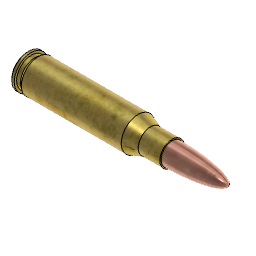
7-62x51mm_FMJ_mk1_v1 (Autodesk Fusion 360 design; units mm, degrees)
Autodesk Fusion 360 part; units mm, degrees
sketch "スケッチ1" plane through (0, 0, 0) normal (0, 0, 1) x (1, 0, 0)
  line L0 (0, 0) -> (71.12, 0)
  line L1 (0.458, 6.007) -> (0.458, -6.007) construction
  line L2 (0, 5.549) -> (0, -5.549)
  line L3 (0.458, 6.007) -> (0, 5.549)
  line L4 (1.372, 5.1945) -> (1.372, -5.1945) construction
  line L5 (0.458, -6.007) -> (1.372, -6.007)
  line L6 (0, -5.549) -> (0.458, -6.007)
  line L7 (0.458, 6.007) -> (1.372, 6.007)
  line L8 (2.769, -5.1945) -> (2.769, 5.1945) construction
  line L9 (2.769, 5.1945) -> (1.372, 5.1945)
  line L10 (2.769, -5.1945) -> (1.372, -5.1945)
  line L11 (1.372, 6.007) -> (1.372, 5.1945)
  line L12 (1.372, -5.1945) -> (1.372, -6.007)
  line L13 (3.8226, 5.96) -> (3.8226, -5.96) construction
  line L14 (2.769, 5.1945) -> (3.8226, 5.96)
  line L15 (2.769, -5.1945) -> (3.8226, -5.96)
  line L16 (39.1509, 5.96) -> (39.1509, -5.96) construction
  line L17 (3.8226, 5.96) -> (39.1509, 5.96)
  line L18 (3.8226, -5.96) -> (3.8604, -5.96)
  line L19 (3.8604, -5.96) -> (39.1509, -5.96)
  line L20 (43.54, 4.3625) -> (43.54, -4.3625) construction
  line L21 (43.54, 4.3625) -> (39.1509, 5.96)
  line L22 (43.54, -4.3625) -> (39.1509, -5.96)
  line L23 (51.181, 4.3625) -> (51.181, -4.3625)
  line L24 (43.54, 4.3625) -> (51.181, 4.3625)
  line L25 (43.54, -4.3625) -> (51.181, -4.3625)
  ellipse E0 centre (51, 0) end of major axis (71.12, 0) minor radius 3.915
  line L26 (30.88, 0) -> (71.12, 0) construction
  line L27 (51, -3.915) -> (51, 3.915) construction
  dimension "d1" = 71.12
  dimension "d2" = 12.014
  dimension "d3" = 0.458
  dimension "d4" = 45
  dimension "d5" = 1.372
  dimension "d7" = 10.389
  dimension "d8" = 1.397
  dimension "d9" = 11.92
  dimension "d11" = 11.92
  dimension "d13" = 8.725
  dimension "d15" = 51.181
  dimension "d36" = 36
  dimension "d39" = 20
  dimension "d40" = 43.54
  dimension "d41" = 7.83
  constraint coincident L0.start origin
  constraint horizontal L0
  constraint perpendicular L0 L1
  constraint symmetric L0 L1.start L1.end
  constraint perpendicular L0 L2
  constraint midpoint L0.start L2
  constraint perpendicular L0 L4
  constraint perpendicular L4 L7
  constraint perpendicular L4 L5
  constraint perpendicular L0 L8
  constraint symmetric L0 L8.start L8.end
  constraint perpendicular L4 L9
  constraint perpendicular L8 L10
  constraint perpendicular L0 L11
  constraint perpendicular L0 L12
  constraint perpendicular L0 L13
  constraint symmetric L0 L13.start L13.end
  constraint perpendicular L0 L16
  constraint symmetric L0 L16.start L16.end
  constraint perpendicular L13 L18
  constraint perpendicular L0 L20
  constraint symmetric L0 L20.start L20.end
  constraint perpendicular L0 L23
  constraint perpendicular L23 L24
  constraint perpendicular L23 L25
  constraint coincident E0 L26.start
  constraint coincident E0 L0.end
  constraint coincident E0 L27.start
  constraint coincident E0 L27.end
  constraint coincident L0 E0.centre
  constraint coincident L0.end L26.end
  measures "d1" distance of L0.start L0.end
  measures "d2" distance of L1.start L1.end
  measures "d3" distance of L1 L2
  measures "d4" angle of L1 L3
  measures "d5" distance of L2 L4
  measures "d7" distance of L8.start L8.end
  measures "d8" distance of L4 L8
  measures "d9" distance of L13.start L13.end
  measures "d11" distance of L16.start L16.end
  measures "d13" distance of L20.start L20.end
  measures "d15" distance of L2 L23
  measures "d36" angle of L0 L14
  measures "d39" angle of L0 L21
  measures "d40" distance of L2 L20
revolve "回転4" add sketch "スケッチ1" angle 360 about axis through (0, 0, 0) along (1, 0, 0) contours L0 L2 L3 L7 L9 L11 L14 L17 L21 L23 L24 E0 | L0 L23 E0 picked at (41.0352, 1.1341) makes body 1
revolve "回転5" add sketch "スケッチ1" angle 360 about axis through (0, 0, 0) along (1, 0, 0) separate body contours L0 L23 E0 picked at (62.5034, 0.9239) makes body 2
sketch "スケッチ5" plane through (51.181, 0, 0) normal (1, 0, 0) x (0, 1, 0)
  circle A0 centre (0, 0) radius 4.3625
  circle A1 centre (0, 0) radius 3.5
  dimension "d45" = 7
  constraint coincident A0.centre A1.centre
  measures "d45" diameter of A1
extrude "押し出し6" cut sketch "スケッチ5" against normal blind 40 contours A1 bodies 1
extrude "押し出し7" add sketch "スケッチ5" against normal blind 5 contours A1 bodies 2
